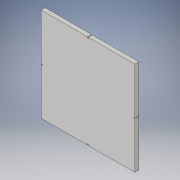
# Autodesk Inventor part: aruco_plate
Saved by Autodesk Inventor 2019 (Build 230136000, 136)
## iProperties
Created: 2024-08-28
Part Number: aruco_plate
Material: Generisch
Document SubType Name: Modeling
Designer: nic
Density: 1 g/cm^3
Appearance: Vorgabe
Author: nic
Autodesk Inventor part; units mm, degrees
ref_plane "YZ Plane" through (0, 0, 0) normal (1, 0, 0) x (0, 1, 0)
ref_plane "XZ Plane" through (0, 0, 0) normal (0, 1, 0) x (-1, 0, 0)
ref_plane "XY Plane" through (0, 0, 0) normal (0, 0, 1) x (1, 0, 0)
sketch "Skizze1" plane through (0, 0, 0) normal (0, 0, 1) x (1, 0, 0)
  line L0 (-34.5, 34.5) -> (34.5, 34.5)
  line L1 (34.5, 34.5) -> (34.5, -34.5)
  line L2 (34.5, -34.5) -> (-34.5, -34.5)
  line L3 (-34.5, -34.5) -> (-34.5, 34.5)
  line L4 (-34.5, 34.5) -> (34.5, -34.5) construction
  line L5 (34.5, 34.5) -> (-34.5, -34.5) construction
  point P0 (0, 0)
  dimension "d0" = 69
  dimension "d1" = 69
  constraints: 12 end point, 2 midpoint, 2 parallel, 1 horizontal, 1 perpendicular
  measures "d0" distance of L1.end L2.end
  measures "d1" distance of L0.end L1.end
extrude "Extrusion1" add sketch "Skizze1" along normal blind 3
sketch "Skizze2" plane through (0, 0, 0) normal (0, 0, -1) x (-1, 0, 0)
  line L0 (34.5, 34.5) -> (-34.5, 34.5) construction
  line L1 (-34.5, 34.5) -> (-34.5, -34.5) construction
  line L2 (-34.5, -34.5) -> (34.5, -34.5) construction
  line L3 (34.5, -34.5) -> (34.5, 34.5) construction
  line L4 (-0.25, -36.2092) -> (0.25, -36.2092) construction
  line L5 (0.25, -36.2092) -> (0.25, 36.2092) construction
  line L6 (0.25, 36.2092) -> (-0.25, 36.2092) construction
  line L7 (-0.25, 36.2092) -> (-0.25, -36.2092) construction
  line L8 (-0.25, -36.2092) -> (0.25, 36.2092) construction
  line L9 (0.25, -36.2092) -> (-0.25, 36.2092) construction
  line L10 (-34.5, -34.5) -> (-34.5, 34.5) construction
  line L11 (34.5, -0.25) -> (-34.5, -0.25) construction
  line L12 (-34.5, -0.25) -> (-34.5, 0.25) construction
  line L13 (-34.5, 0.25) -> (34.5, 0.25) construction
  line L14 (34.5, 0.25) -> (34.5, -0.25) construction
  line L15 (34.5, -0.25) -> (-34.5, 0.25) construction
  line L16 (-34.5, -0.25) -> (34.5, 0.25) construction
  line L17 (-0.2382, 34.5) -> (0.2313, 34.5)
  line L18 (0.2313, 34.5) -> (0.2313, 33.5)
  line L19 (0.2313, 33.5) -> (-0.2382, 33.5)
  line L20 (-0.2382, 33.5) -> (-0.2382, 34.5)
  line L21 (-34.5, 0.25) -> (-33.5, 0.25)
  line L22 (-33.5, 0.25) -> (-33.5, -0.2428)
  line L23 (-33.5, -0.2428) -> (-34.5, -0.2428)
  line L24 (-34.5, -0.2428) -> (-34.5, 0.25)
  line L25 (34.5, -34.5) -> (-34.5, -34.5) projected
  line L26 (-0.25, -34.5) -> (0.25, -34.5)
  line L27 (0.25, -34.5) -> (0.25, -33.5)
  line L28 (0.25, -33.5) -> (-0.25, -33.5)
  line L29 (-0.25, -33.5) -> (-0.25, -34.5)
  line L30 (34.5, 0.25) -> (33.5, 0.25)
  line L31 (33.5, 0.25) -> (33.5, -0.2428)
  line L32 (33.5, -0.2428) -> (34.5, -0.2428)
  line L33 (34.5, -0.2428) -> (34.5, 0.25)
  point P0 (0, 0)
  dimension "d4" = 0.5
  dimension "d5" = 0.5
  dimension "d6" = 1
  dimension "d7" = 1
  dimension "d8" = 1
  dimension "d9" = 1
  constraints: 56 end point, 12 parallel, 9 point on line, 6 horizontal, 6 perpendicular, 4 midpoint
  measures "d4" distance of L6.end L5.end
  measures "d5" distance of L11.end L12.end
  measures "d6" distance of L17.end L18.end
  measures "d7" distance of L22.end L23.end
  measures "d8" distance of L27.end L26.end
  measures "d9" distance of L32.end L31.end
extrude "Extrusion2" cut sketch "Skizze2" against normal through all
sketch "Skizze3" plane through (0, 0, 0) normal (0, 0, -1) x (-1, 0, 0)
  line L0 (13.5227, 32.2329) -> (32.4466, 32.2329) construction
  line L1 (32.4466, 32.2329) -> (32.4466, 28.5854) construction
  line L2 (32.4466, 28.5854) -> (13.5227, 28.5854) construction
  line L3 (13.5227, 28.5854) -> (13.5227, 32.2329) construction
  line L4 (14.0662, 25.0881) -> (28.9058, 25.0881) construction
  line L5 (28.9058, 25.0881) -> (28.9058, 21.4406) construction
  line L6 (28.9058, 21.4406) -> (14.0662, 21.4406) construction
  line L7 (14.0662, 21.4406) -> (14.0662, 25.0881) construction
  spline S0 degree 2 poles (16.4431, 22.6261) (16.4431, 22.3737) (16.2814, 21.9426) (16.1339, 21.7838) knots 0 0 0 1 2 2 2
  spline S1 degree 2 poles (16.1339, 21.7838) (15.9864, 21.6249) (15.5468, 21.4406) (15.2745, 21.4406) knots 0 0 0 1 2 2 2
  spline S2 degree 2 poles (15.2745, 21.4406) (15.0249, 21.4406) (14.5371, 21.5512) (14.3584, 21.6391) knots 0 0 0 1 2 2 2
  line L8 (14.3584, 21.6391) -> (14.3584, 22.1355)
  line L9 (14.3584, 22.1355) -> (14.3924, 22.1355)
  spline S3 degree 2 poles (14.3924, 22.1355) (14.4463, 22.0958) (14.6477, 21.9937) (14.7696, 21.9483) knots 0 0 0 1 2 2 2
  spline S4 degree 2 poles (14.7696, 21.9483) (14.9086, 21.9001) (15.1384, 21.8462) (15.283, 21.8462) knots 0 0 0 1 2 2 2
  spline S5 degree 2 poles (15.283, 21.8462) (15.4248, 21.8462) (15.6914, 21.9483) (15.7879, 22.0589) knots 0 0 0 1 2 2 2
  spline S6 degree 2 poles (15.7879, 22.0589) (15.8758, 22.1638) (15.9666, 22.4418) (15.9666, 22.629) knots 0 0 0 1 2 2 2
  spline S7 degree 2 poles (15.9666, 22.629) (15.9666, 22.8162) (15.8645, 23.0544) (15.768, 23.1338) knots 0 0 0 1 2 2 2
  spline S8 degree 2 poles (15.768, 23.1338) (15.6687, 23.2218) (15.3738, 23.2955) (15.1951, 23.2955) knots 0 0 0 1 2 2 2
  spline S9 degree 2 poles (15.1951, 23.2955) (15.0022, 23.2955) (14.6193, 23.236) (14.503, 23.2104) knots 0 0 0 1 2 2 2
  line L10 (14.503, 23.2104) -> (14.503, 25.0143)
  line L11 (14.503, 25.0143) -> (16.4232, 25.0143)
  line L12 (16.4232, 25.0143) -> (16.4232, 24.6031)
  line L13 (16.4232, 24.6031) -> (14.954, 24.6031)
  line L14 (14.954, 24.6031) -> (14.954, 23.6699)
  spline S10 degree 2 poles (14.954, 23.6699) (15.0391, 23.6813) (15.2036, 23.6898) (15.2717, 23.6898) knots 0 0 0 1 2 2 2
  spline S11 degree 2 poles (15.2717, 23.6898) (15.5411, 23.6898) (15.9127, 23.6018) (16.0828, 23.4714) knots 0 0 0 1 2 2 2
  spline S12 degree 2 poles (16.0828, 23.4714) (16.2559, 23.3409) (16.4431, 22.9438) (16.4431, 22.6261) knots 0 0 0 1 2 2 2
  spline S13 degree 2 poles (17.8924, 24.6825) (17.7648, 24.6825) (17.5123, 24.6201) (17.3904, 24.5719) knots 0 0 0 1 2 2 2
  spline S14 degree 2 poles (17.3904, 24.5719) (17.2769, 24.5236) (17.1096, 24.4215) (17.0444, 24.3761) knots 0 0 0 1 2 2 2
  line L15 (17.0444, 24.3761) -> (17.016, 24.3761)
  line L16 (17.016, 24.3761) -> (17.016, 24.8725)
  spline S15 degree 2 poles (17.016, 24.8725) (17.1692, 24.9548) (17.6939, 25.0881) (17.9293, 25.0881) knots 0 0 0 1 2 2 2
  spline S16 degree 2 poles (17.9293, 25.0881) (18.1675, 25.0881) (18.5221, 24.9916) (18.6667, 24.8895) knots 0 0 0 1 2 2 2
  spline S17 degree 2 poles (18.6667, 24.8895) (18.8199, 24.7789) (18.9787, 24.4584) (18.9787, 24.2428) knots 0 0 0 1 2 2 2
  spline S18 degree 2 poles (18.9787, 24.2428) (18.9787, 23.9535) (18.5986, 23.5167) (18.332, 23.46) knots 0 0 0 1 2 2 2
  line L17 (18.332, 23.46) -> (18.332, 23.426)
  spline S19 degree 2 poles (18.332, 23.426) (18.4427, 23.4033) (18.6951, 23.3012) (18.8029, 23.1991) knots 0 0 0 1 2 2 2
  spline S20 degree 2 poles (18.8029, 23.1991) (18.9106, 23.0998) (19.0468, 22.7821) (19.0468, 22.5524) knots 0 0 0 1 2 2 2
  spline S21 degree 2 poles (19.0468, 22.5524) (19.0468, 22.317) (18.8851, 21.9171) (18.7376, 21.7639) knots 0 0 0 1 2 2 2
  spline S22 degree 2 poles (18.7376, 21.7639) (18.5845, 21.6051) (18.1505, 21.4406) (17.8754, 21.4406) knots 0 0 0 1 2 2 2
  spline S23 degree 2 poles (17.8754, 21.4406) (17.6116, 21.4406) (17.0954, 21.5682) (16.9196, 21.6561) knots 0 0 0 1 2 2 2
  line L18 (16.9196, 21.6561) -> (16.9196, 22.1525)
  line L19 (16.9196, 22.1525) -> (16.9536, 22.1525)
  spline S24 degree 2 poles (16.9536, 22.1525) (17.1011, 22.0447) (17.6003, 21.8462) (17.847, 21.8462) knots 0 0 0 1 2 2 2
  spline S25 degree 2 poles (17.847, 21.8462) (17.9917, 21.8462) (18.281, 21.9369) (18.3774, 22.0419) knots 0 0 0 1 2 2 2
  spline S26 degree 2 poles (18.3774, 22.0419) (18.471, 22.1468) (18.5703, 22.3964) (18.5703, 22.5864) knots 0 0 0 1 2 2 2
  spline S27 degree 2 poles (18.5703, 22.5864) (18.5703, 22.7765) (18.4597, 23.0232) (18.3604, 23.0941) knots 0 0 0 1 2 2 2
  spline S28 degree 2 poles (18.3604, 23.0941) (18.2611, 23.165) (17.9917, 23.2189) (17.8328, 23.2189) knots 0 0 0 1 2 2 2
  line L20 (17.8328, 23.2189) -> (17.6343, 23.2189)
  line L21 (17.6343, 23.2189) -> (17.6343, 23.6075)
  line L22 (17.6343, 23.6075) -> (17.7903, 23.6075)
  spline S29 degree 2 poles (17.7903, 23.6075) (18.1051, 23.6075) (18.5022, 23.9082) (18.5022, 24.1946) knots 0 0 0 1 2 2 2
  spline S30 degree 2 poles (18.5022, 24.1946) (18.5022, 24.3279) (18.4001, 24.518) (18.3179, 24.5747) knots 0 0 0 1 2 2 2
  spline S31 degree 2 poles (18.3179, 24.5747) (18.2299, 24.6342) (18.0144, 24.6825) (17.8924, 24.6825) knots 0 0 0 1 2 2 2
  line L23 (21.6789, 21.5143) -> (21.1371, 21.5143)
  line L24 (21.1371, 21.5143) -> (20.499, 22.5013)
  line L25 (20.499, 22.5013) -> (19.8438, 21.5143)
  line L26 (19.8438, 21.5143) -> (19.3418, 21.5143)
  line L27 (19.3418, 21.5143) -> (20.2522, 22.8162)
  line L28 (20.2522, 22.8162) -> (19.3503, 24.1407)
  line L29 (19.3503, 24.1407) -> (19.892, 24.1407)
  line L30 (19.892, 24.1407) -> (20.5273, 23.1622)
  line L31 (20.5273, 23.1622) -> (21.1769, 24.1407)
  line L32 (21.1769, 24.1407) -> (21.6789, 24.1407)
  line L33 (21.6789, 24.1407) -> (20.7741, 22.8445)
  line L34 (20.7741, 22.8445) -> (21.6789, 21.5143)
  spline S32 degree 2 poles (24.0784, 22.6261) (24.0784, 22.3737) (23.9167, 21.9426) (23.7692, 21.7838) knots 0 0 0 1 2 2 2
  spline S33 degree 2 poles (23.7692, 21.7838) (23.6217, 21.6249) (23.1821, 21.4406) (22.9098, 21.4406) knots 0 0 0 1 2 2 2
  spline S34 degree 2 poles (22.9098, 21.4406) (22.6602, 21.4406) (22.1724, 21.5512) (21.9937, 21.6391) knots 0 0 0 1 2 2 2
  line L35 (21.9937, 21.6391) -> (21.9937, 22.1355)
  line L36 (21.9937, 22.1355) -> (22.0277, 22.1355)
  spline S35 degree 2 poles (22.0277, 22.1355) (22.0816, 22.0958) (22.283, 21.9937) (22.405, 21.9483) knots 0 0 0 1 2 2 2
  spline S36 degree 2 poles (22.405, 21.9483) (22.5439, 21.9001) (22.7737, 21.8462) (22.9183, 21.8462) knots 0 0 0 1 2 2 2
  spline S37 degree 2 poles (22.9183, 21.8462) (23.0602, 21.8462) (23.3268, 21.9483) (23.4232, 22.0589) knots 0 0 0 1 2 2 2
  spline S38 degree 2 poles (23.4232, 22.0589) (23.5111, 22.1638) (23.6019, 22.4418) (23.6019, 22.629) knots 0 0 0 1 2 2 2
  spline S39 degree 2 poles (23.6019, 22.629) (23.6019, 22.8162) (23.4998, 23.0544) (23.4033, 23.1338) knots 0 0 0 1 2 2 2
  spline S40 degree 2 poles (23.4033, 23.1338) (23.3041, 23.2218) (23.0091, 23.2955) (22.8304, 23.2955) knots 0 0 0 1 2 2 2
  spline S41 degree 2 poles (22.8304, 23.2955) (22.6375, 23.2955) (22.2546, 23.236) (22.1384, 23.2104) knots 0 0 0 1 2 2 2
  line L37 (22.1384, 23.2104) -> (22.1384, 25.0143)
  line L38 (22.1384, 25.0143) -> (24.0585, 25.0143)
  line L39 (24.0585, 25.0143) -> (24.0585, 24.6031)
  line L40 (24.0585, 24.6031) -> (22.5893, 24.6031)
  line L41 (22.5893, 24.6031) -> (22.5893, 23.6699)
  spline S42 degree 2 poles (22.5893, 23.6699) (22.6744, 23.6813) (22.8389, 23.6898) (22.907, 23.6898) knots 0 0 0 1 2 2 2
  spline S43 degree 2 poles (22.907, 23.6898) (23.1764, 23.6898) (23.548, 23.6018) (23.7182, 23.4714) knots 0 0 0 1 2 2 2
  spline S44 degree 2 poles (23.7182, 23.4714) (23.8912, 23.3409) (24.0784, 22.9438) (24.0784, 22.6261) knots 0 0 0 1 2 2 2
  spline S45 degree 2 poles (25.5277, 24.6825) (25.4001, 24.6825) (25.1477, 24.6201) (25.0257, 24.5719) knots 0 0 0 1 2 2 2
  spline S46 degree 2 poles (25.0257, 24.5719) (24.9123, 24.5236) (24.7449, 24.4215) (24.6797, 24.3761) knots 0 0 0 1 2 2 2
  line L42 (24.6797, 24.3761) -> (24.6513, 24.3761)
  line L43 (24.6513, 24.3761) -> (24.6513, 24.8725)
  spline S47 degree 2 poles (24.6513, 24.8725) (24.8045, 24.9548) (25.3292, 25.0881) (25.5646, 25.0881) knots 0 0 0 1 2 2 2
  spline S48 degree 2 poles (25.5646, 25.0881) (25.8029, 25.0881) (26.1574, 24.9916) (26.3021, 24.8895) knots 0 0 0 1 2 2 2
  spline S49 degree 2 poles (26.3021, 24.8895) (26.4552, 24.7789) (26.614, 24.4584) (26.614, 24.2428) knots 0 0 0 1 2 2 2
  spline S50 degree 2 poles (26.614, 24.2428) (26.614, 23.9535) (26.234, 23.5167) (25.9674, 23.46) knots 0 0 0 1 2 2 2
  line L44 (25.9674, 23.46) -> (25.9674, 23.426)
  spline S51 degree 2 poles (25.9674, 23.426) (26.078, 23.4033) (26.3304, 23.3012) (26.4382, 23.1991) knots 0 0 0 1 2 2 2
  spline S52 degree 2 poles (26.4382, 23.1991) (26.546, 23.0998) (26.6821, 22.7821) (26.6821, 22.5524) knots 0 0 0 1 2 2 2
  spline S53 degree 2 poles (26.6821, 22.5524) (26.6821, 22.317) (26.5204, 21.9171) (26.373, 21.7639) knots 0 0 0 1 2 2 2
  spline S54 degree 2 poles (26.373, 21.7639) (26.2198, 21.6051) (25.7858, 21.4406) (25.5107, 21.4406) knots 0 0 0 1 2 2 2
  spline S55 degree 2 poles (25.5107, 21.4406) (25.2469, 21.4406) (24.7307, 21.5682) (24.5549, 21.6561) knots 0 0 0 1 2 2 2
  line L45 (24.5549, 21.6561) -> (24.5549, 22.1525)
  line L46 (24.5549, 22.1525) -> (24.5889, 22.1525)
  spline S56 degree 2 poles (24.5889, 22.1525) (24.7364, 22.0447) (25.2356, 21.8462) (25.4824, 21.8462) knots 0 0 0 1 2 2 2
  spline S57 degree 2 poles (25.4824, 21.8462) (25.627, 21.8462) (25.9163, 21.9369) (26.0127, 22.0419) knots 0 0 0 1 2 2 2
  spline S58 degree 2 poles (26.0127, 22.0419) (26.1063, 22.1468) (26.2056, 22.3964) (26.2056, 22.5864) knots 0 0 0 1 2 2 2
  spline S59 degree 2 poles (26.2056, 22.5864) (26.2056, 22.7765) (26.095, 23.0232) (25.9957, 23.0941) knots 0 0 0 1 2 2 2
  spline S60 degree 2 poles (25.9957, 23.0941) (25.8965, 23.165) (25.627, 23.2189) (25.4682, 23.2189) knots 0 0 0 1 2 2 2
  line L47 (25.4682, 23.2189) -> (25.2696, 23.2189)
  line L48 (25.2696, 23.2189) -> (25.2696, 23.6075)
  line L49 (25.2696, 23.6075) -> (25.4256, 23.6075)
  spline S61 degree 2 poles (25.4256, 23.6075) (25.7405, 23.6075) (26.1375, 23.9082) (26.1375, 24.1946) knots 0 0 0 1 2 2 2
  spline S62 degree 2 poles (26.1375, 24.1946) (26.1375, 24.3279) (26.0354, 24.518) (25.9532, 24.5747) knots 0 0 0 1 2 2 2
  spline S63 degree 2 poles (25.9532, 24.5747) (25.8653, 24.6342) (25.6497, 24.6825) (25.5277, 24.6825) knots 0 0 0 1 2 2 2
  spline S64 degree 2 poles (15.9903, 29.7937) (15.9903, 29.5242) (15.8116, 29.0676) (15.6613, 28.9144) knots 0 0 0 1 2 2 2
  spline S65 degree 2 poles (15.6613, 28.9144) (15.5053, 28.7527) (15.1139, 28.5854) (14.8785, 28.5854) knots 0 0 0 1 2 2 2
  spline S66 degree 2 poles (14.8785, 28.5854) (14.6431, 28.5854) (14.2545, 28.7442) (14.107, 28.9031) knots 0 0 0 1 2 2 2
  spline S67 degree 2 poles (14.107, 28.9031) (13.9255, 29.0931) (13.7213, 29.7313) (13.7213, 30.1964) knots 0 0 0 1 2 2 2
  spline S68 degree 2 poles (13.7213, 30.1964) (13.7213, 30.6531) (13.9085, 31.3877) (14.1042, 31.66) knots 0 0 0 1 2 2 2
  spline S69 degree 2 poles (14.1042, 31.66) (14.2942, 31.9266) (14.8955, 32.2244) (15.2898, 32.2244) knots 0 0 0 1 2 2 2
  spline S70 degree 2 poles (15.2898, 32.2244) (15.406, 32.2244) (15.6103, 32.2017) (15.6868, 32.1762) knots 0 0 0 1 2 2 2
  line L50 (15.6868, 32.1762) -> (15.6868, 31.7252)
  line L51 (15.6868, 31.7252) -> (15.667, 31.7252)
  spline S71 degree 2 poles (15.667, 31.7252) (15.6018, 31.7592) (15.3635, 31.8188) (15.2274, 31.8188) knots 0 0 0 1 2 2 2
  spline S72 degree 2 poles (15.2274, 31.8188) (14.7906, 31.8188) (14.2545, 31.2288) (14.2035, 30.6502) knots 0 0 0 1 2 2 2
  spline S73 degree 2 poles (14.2035, 30.6502) (14.3708, 30.7665) (14.7225, 30.8942) (14.9324, 30.8942) knots 0 0 0 1 2 2 2
  spline S74 degree 2 poles (14.9324, 30.8942) (15.1366, 30.8942) (15.4429, 30.8119) (15.6103, 30.6871) knots 0 0 0 1 2 2 2
  spline S75 degree 2 poles (15.6103, 30.6871) (15.8031, 30.5425) (15.9903, 30.0943) (15.9903, 29.7937) knots 0 0 0 1 2 2 2
  spline S76 degree 2 poles (15.5138, 29.7738) (15.5138, 29.9894) (15.4004, 30.2815) (15.2756, 30.3836) knots 0 0 0 1 2 2 2
  spline S77 degree 2 poles (15.2756, 30.3836) (15.182, 30.4574) (14.9494, 30.5056) (14.8274, 30.5056) knots 0 0 0 1 2 2 2
  spline S78 degree 2 poles (14.8274, 30.5056) (14.6629, 30.5056) (14.3538, 30.4063) (14.2035, 30.3127) knots 0 0 0 1 2 2 2
  spline S79 degree 2 poles (14.2035, 30.3127) (14.2006, 30.2617) (14.1949, 30.1652) (14.1949, 30.0915) knots 0 0 0 1 2 2 2
  spline S80 degree 2 poles (14.1949, 30.0915) (14.1949, 29.7284) (14.3368, 29.2831) (14.4445, 29.1668) knots 0 0 0 1 2 2 2
  spline S81 degree 2 poles (14.4445, 29.1668) (14.5438, 29.0562) (14.7594, 28.9683) (14.8813, 28.9683) knots 0 0 0 1 2 2 2
  spline S82 degree 2 poles (14.8813, 28.9683) (15.165, 28.9683) (15.5138, 29.3711) (15.5138, 29.7738) knots 0 0 0 1 2 2 2
  spline S83 degree 2 poles (16.308, 31.0218) (16.308, 31.2912) (16.4838, 31.7394) (16.637, 31.901) knots 0 0 0 1 2 2 2
  spline S84 degree 2 poles (16.637, 31.901) (16.7817, 32.057) (17.2043, 32.2301) (17.4198, 32.2301) knots 0 0 0 1 2 2 2
  spline S85 degree 2 poles (17.4198, 32.2301) (17.6609, 32.2301) (18.0523, 32.0684) (18.197, 31.9152) knots 0 0 0 1 2 2 2
  spline S86 degree 2 poles (18.197, 31.9152) (18.3785, 31.7224) (18.577, 31.0984) (18.577, 30.619) knots 0 0 0 1 2 2 2
  spline S87 degree 2 poles (18.577, 30.619) (18.577, 30.1851) (18.3813, 29.4079) (18.1913, 29.1498) knots 0 0 0 1 2 2 2
  spline S88 degree 2 poles (18.1913, 29.1498) (17.9899, 28.8775) (17.4227, 28.5911) (17.0086, 28.5911) knots 0 0 0 1 2 2 2
  spline S89 degree 2 poles (17.0086, 28.5911) (16.915, 28.5911) (16.7022, 28.6109) (16.6115, 28.6393) knots 0 0 0 1 2 2 2
  line L52 (16.6115, 28.6393) -> (16.6115, 29.0903)
  line L53 (16.6115, 29.0903) -> (16.6342, 29.0903)
  spline S90 degree 2 poles (16.6342, 29.0903) (16.6937, 29.0562) (16.9433, 28.9967) (17.071, 28.9967) knots 0 0 0 1 2 2 2
  spline S91 degree 2 poles (17.071, 28.9967) (17.5304, 28.9967) (18.0552, 29.6036) (18.092, 30.1652) knots 0 0 0 1 2 2 2
  spline S92 degree 2 poles (18.092, 30.1652) (17.9048, 30.0376) (17.5645, 29.9213) (17.3631, 29.9213) knots 0 0 0 1 2 2 2
  spline S93 degree 2 poles (17.3631, 29.9213) (17.1702, 29.9213) (16.8497, 30.0064) (16.6881, 30.1284) knots 0 0 0 1 2 2 2
  spline S94 degree 2 poles (16.6881, 30.1284) (16.5009, 30.273) (16.308, 30.7126) (16.308, 31.0218) knots 0 0 0 1 2 2 2
  spline S95 degree 2 poles (18.1034, 30.724) (18.1034, 31.0785) (17.9729, 31.5267) (17.8566, 31.6486) knots 0 0 0 1 2 2 2
  spline S96 degree 2 poles (17.8566, 31.6486) (17.7545, 31.7621) (17.5418, 31.8472) (17.417, 31.8472) knots 0 0 0 1 2 2 2
  spline S97 degree 2 poles (17.417, 31.8472) (17.1277, 31.8472) (16.7845, 31.4331) (16.7845, 31.0416) knots 0 0 0 1 2 2 2
  spline S98 degree 2 poles (16.7845, 31.0416) (16.7845, 30.8204) (16.8979, 30.5339) (17.0227, 30.4318) knots 0 0 0 1 2 2 2
  spline S99 degree 2 poles (17.0227, 30.4318) (17.1135, 30.3581) (17.3376, 30.3099) (17.468, 30.3099) knots 0 0 0 1 2 2 2
  spline S100 degree 2 poles (17.468, 30.3099) (17.6184, 30.3099) (17.9644, 30.4148) (18.0949, 30.5027) knots 0 0 0 1 2 2 2
  spline S101 degree 2 poles (18.0949, 30.5027) (18.0977, 30.5368) (18.1034, 30.6531) (18.1034, 30.724) knots 0 0 0 1 2 2 2
  line L54 (21.1354, 28.6591) -> (20.5936, 28.6591)
  line L55 (20.5936, 28.6591) -> (19.9555, 29.6462)
  line L56 (19.9555, 29.6462) -> (19.3003, 28.6591)
  line L57 (19.3003, 28.6591) -> (18.7983, 28.6591)
  line L58 (18.7983, 28.6591) -> (19.7087, 29.961)
  line L59 (19.7087, 29.961) -> (18.8068, 31.2856)
  line L60 (18.8068, 31.2856) -> (19.3485, 31.2856)
  line L61 (19.3485, 31.2856) -> (19.9838, 30.307)
  line L62 (19.9838, 30.307) -> (20.6334, 31.2856)
  line L63 (20.6334, 31.2856) -> (21.1354, 31.2856)
  line L64 (21.1354, 31.2856) -> (20.2306, 29.9894)
  line L65 (20.2306, 29.9894) -> (21.1354, 28.6591)
  spline S102 degree 2 poles (23.6257, 29.7937) (23.6257, 29.5242) (23.447, 29.0676) (23.2966, 28.9144) knots 0 0 0 1 2 2 2
  spline S103 degree 2 poles (23.2966, 28.9144) (23.1406, 28.7527) (22.7492, 28.5854) (22.5138, 28.5854) knots 0 0 0 1 2 2 2
  spline S104 degree 2 poles (22.5138, 28.5854) (22.2784, 28.5854) (21.8898, 28.7442) (21.7424, 28.9031) knots 0 0 0 1 2 2 2
  spline S105 degree 2 poles (21.7424, 28.9031) (21.5608, 29.0931) (21.3566, 29.7313) (21.3566, 30.1964) knots 0 0 0 1 2 2 2
  spline S106 degree 2 poles (21.3566, 30.1964) (21.3566, 30.6531) (21.5438, 31.3877) (21.7395, 31.66) knots 0 0 0 1 2 2 2
  spline S107 degree 2 poles (21.7395, 31.66) (21.9295, 31.9266) (22.5308, 32.2244) (22.9251, 32.2244) knots 0 0 0 1 2 2 2
  spline S108 degree 2 poles (22.9251, 32.2244) (23.0414, 32.2244) (23.2456, 32.2017) (23.3222, 32.1762) knots 0 0 0 1 2 2 2
  line L66 (23.3222, 32.1762) -> (23.3222, 31.7252)
  line L67 (23.3222, 31.7252) -> (23.3023, 31.7252)
  spline S109 degree 2 poles (23.3023, 31.7252) (23.2371, 31.7592) (22.9988, 31.8188) (22.8627, 31.8188) knots 0 0 0 1 2 2 2
  spline S110 degree 2 poles (22.8627, 31.8188) (22.4259, 31.8188) (21.8898, 31.2288) (21.8388, 30.6502) knots 0 0 0 1 2 2 2
  spline S111 degree 2 poles (21.8388, 30.6502) (22.0061, 30.7665) (22.3578, 30.8942) (22.5677, 30.8942) knots 0 0 0 1 2 2 2
  spline S112 degree 2 poles (22.5677, 30.8942) (22.7719, 30.8942) (23.0783, 30.8119) (23.2456, 30.6871) knots 0 0 0 1 2 2 2
  spline S113 degree 2 poles (23.2456, 30.6871) (23.4385, 30.5425) (23.6257, 30.0943) (23.6257, 29.7937) knots 0 0 0 1 2 2 2
  spline S114 degree 2 poles (23.1492, 29.7738) (23.1492, 29.9894) (23.0357, 30.2815) (22.9109, 30.3836) knots 0 0 0 1 2 2 2
  spline S115 degree 2 poles (22.9109, 30.3836) (22.8173, 30.4574) (22.5847, 30.5056) (22.4628, 30.5056) knots 0 0 0 1 2 2 2
  spline S116 degree 2 poles (22.4628, 30.5056) (22.2983, 30.5056) (21.9891, 30.4063) (21.8388, 30.3127) knots 0 0 0 1 2 2 2
  spline S117 degree 2 poles (21.8388, 30.3127) (21.8359, 30.2617) (21.8303, 30.1652) (21.8303, 30.0915) knots 0 0 0 1 2 2 2
  spline S118 degree 2 poles (21.8303, 30.0915) (21.8303, 29.7284) (21.9721, 29.2831) (22.0799, 29.1668) knots 0 0 0 1 2 2 2
  spline S119 degree 2 poles (22.0799, 29.1668) (22.1791, 29.0562) (22.3947, 28.9683) (22.5167, 28.9683) knots 0 0 0 1 2 2 2
  spline S120 degree 2 poles (22.5167, 28.9683) (22.8003, 28.9683) (23.1492, 29.3711) (23.1492, 29.7738) knots 0 0 0 1 2 2 2
  spline S121 degree 2 poles (23.9433, 31.0218) (23.9433, 31.2912) (24.1192, 31.7394) (24.2723, 31.901) knots 0 0 0 1 2 2 2
  spline S122 degree 2 poles (24.2723, 31.901) (24.417, 32.057) (24.8396, 32.2301) (25.0552, 32.2301) knots 0 0 0 1 2 2 2
  spline S123 degree 2 poles (25.0552, 32.2301) (25.2962, 32.2301) (25.6877, 32.0684) (25.8323, 31.9152) knots 0 0 0 1 2 2 2
  spline S124 degree 2 poles (25.8323, 31.9152) (26.0138, 31.7224) (26.2124, 31.0984) (26.2124, 30.619) knots 0 0 0 1 2 2 2
  spline S125 degree 2 poles (26.2124, 30.619) (26.2124, 30.1851) (26.0167, 29.4079) (25.8266, 29.1498) knots 0 0 0 1 2 2 2
  spline S126 degree 2 poles (25.8266, 29.1498) (25.6253, 28.8775) (25.058, 28.5911) (24.6439, 28.5911) knots 0 0 0 1 2 2 2
  spline S127 degree 2 poles (24.6439, 28.5911) (24.5503, 28.5911) (24.3376, 28.6109) (24.2468, 28.6393) knots 0 0 0 1 2 2 2
  line L68 (24.2468, 28.6393) -> (24.2468, 29.0903)
  line L69 (24.2468, 29.0903) -> (24.2695, 29.0903)
  spline S128 degree 2 poles (24.2695, 29.0903) (24.3291, 29.0562) (24.5787, 28.9967) (24.7063, 28.9967) knots 0 0 0 1 2 2 2
  spline S129 degree 2 poles (24.7063, 28.9967) (25.1658, 28.9967) (25.6905, 29.6036) (25.7274, 30.1652) knots 0 0 0 1 2 2 2
  spline S130 degree 2 poles (25.7274, 30.1652) (25.5402, 30.0376) (25.1998, 29.9213) (24.9984, 29.9213) knots 0 0 0 1 2 2 2
  spline S131 degree 2 poles (24.9984, 29.9213) (24.8056, 29.9213) (24.4851, 30.0064) (24.3234, 30.1284) knots 0 0 0 1 2 2 2
  spline S132 degree 2 poles (24.3234, 30.1284) (24.1362, 30.273) (23.9433, 30.7126) (23.9433, 31.0218) knots 0 0 0 1 2 2 2
  spline S133 degree 2 poles (25.7387, 30.724) (25.7387, 31.0785) (25.6082, 31.5267) (25.4919, 31.6486) knots 0 0 0 1 2 2 2
  spline S134 degree 2 poles (25.4919, 31.6486) (25.3898, 31.7621) (25.1771, 31.8472) (25.0523, 31.8472) knots 0 0 0 1 2 2 2
  spline S135 degree 2 poles (25.0523, 31.8472) (24.763, 31.8472) (24.4198, 31.4331) (24.4198, 31.0416) knots 0 0 0 1 2 2 2
  spline S136 degree 2 poles (24.4198, 31.0416) (24.4198, 30.8204) (24.5333, 30.5339) (24.6581, 30.4318) knots 0 0 0 1 2 2 2
  spline S137 degree 2 poles (24.6581, 30.4318) (24.7488, 30.3581) (24.9729, 30.3099) (25.1034, 30.3099) knots 0 0 0 1 2 2 2
  spline S138 degree 2 poles (25.1034, 30.3099) (25.2537, 30.3099) (25.5997, 30.4148) (25.7302, 30.5027) knots 0 0 0 1 2 2 2
  spline S139 degree 2 poles (25.7302, 30.5027) (25.733, 30.5368) (25.7387, 30.6531) (25.7387, 30.724) knots 0 0 0 1 2 2 2
  line L70 (28.7707, 28.6591) -> (28.229, 28.6591)
  line L71 (28.229, 28.6591) -> (27.5908, 29.6462)
  line L72 (27.5908, 29.6462) -> (26.9356, 28.6591)
  line L73 (26.9356, 28.6591) -> (26.4336, 28.6591)
  line L74 (26.4336, 28.6591) -> (27.3441, 29.961)
  line L75 (27.3441, 29.961) -> (26.4421, 31.2856)
  line L76 (26.4421, 31.2856) -> (26.9838, 31.2856)
  line L77 (26.9838, 31.2856) -> (27.6192, 30.307)
  line L78 (27.6192, 30.307) -> (28.2687, 31.2856)
  line L79 (28.2687, 31.2856) -> (28.7707, 31.2856)
  line L80 (28.7707, 31.2856) -> (27.8659, 29.9894)
  line L81 (27.8659, 29.9894) -> (28.7707, 28.6591)
  spline S140 degree 2 poles (29.9932, 31.8273) (29.8655, 31.8273) (29.6131, 31.7649) (29.4911, 31.7167) knots 0 0 0 1 2 2 2
  spline S141 degree 2 poles (29.4911, 31.7167) (29.3777, 31.6685) (29.2103, 31.5664) (29.1451, 31.521) knots 0 0 0 1 2 2 2
  line L82 (29.1451, 31.521) -> (29.1167, 31.521)
  line L83 (29.1167, 31.521) -> (29.1167, 32.0173)
  spline S142 degree 2 poles (29.1167, 32.0173) (29.2699, 32.0996) (29.7946, 32.2329) (30.03, 32.2329) knots 0 0 0 1 2 2 2
  spline S143 degree 2 poles (30.03, 32.2329) (30.2683, 32.2329) (30.6228, 32.1365) (30.7675, 32.0343) knots 0 0 0 1 2 2 2
  spline S144 degree 2 poles (30.7675, 32.0343) (30.9206, 31.9237) (31.0795, 31.6032) (31.0795, 31.3877) knots 0 0 0 1 2 2 2
  spline S145 degree 2 poles (31.0795, 31.3877) (31.0795, 31.0984) (30.6994, 30.6616) (30.4328, 30.6049) knots 0 0 0 1 2 2 2
  line L84 (30.4328, 30.6049) -> (30.4328, 30.5708)
  spline S146 degree 2 poles (30.4328, 30.5708) (30.5434, 30.5481) (30.7958, 30.446) (30.9036, 30.3439) knots 0 0 0 1 2 2 2
  spline S147 degree 2 poles (30.9036, 30.3439) (31.0114, 30.2446) (31.1475, 29.927) (31.1475, 29.6972) knots 0 0 0 1 2 2 2
  spline S148 degree 2 poles (31.1475, 29.6972) (31.1475, 29.4618) (30.9859, 29.0619) (30.8384, 28.9087) knots 0 0 0 1 2 2 2
  spline S149 degree 2 poles (30.8384, 28.9087) (30.6852, 28.7499) (30.2513, 28.5854) (29.9761, 28.5854) knots 0 0 0 1 2 2 2
  spline S150 degree 2 poles (29.9761, 28.5854) (29.7124, 28.5854) (29.1962, 28.713) (29.0203, 28.801) knots 0 0 0 1 2 2 2
  line L85 (29.0203, 28.801) -> (29.0203, 29.2973)
  line L86 (29.0203, 29.2973) -> (29.0543, 29.2973)
  spline S151 degree 2 poles (29.0543, 29.2973) (29.2018, 29.1895) (29.701, 28.991) (29.9478, 28.991) knots 0 0 0 1 2 2 2
  spline S152 degree 2 poles (29.9478, 28.991) (30.0924, 28.991) (30.3817, 29.0818) (30.4782, 29.1867) knots 0 0 0 1 2 2 2
  spline S153 degree 2 poles (30.4782, 29.1867) (30.5718, 29.2916) (30.671, 29.5412) (30.671, 29.7313) knots 0 0 0 1 2 2 2
  spline S154 degree 2 poles (30.671, 29.7313) (30.671, 29.9213) (30.5604, 30.1681) (30.4612, 30.239) knots 0 0 0 1 2 2 2
  spline S155 degree 2 poles (30.4612, 30.239) (30.3619, 30.3099) (30.0924, 30.3638) (29.9336, 30.3638) knots 0 0 0 1 2 2 2
  line L87 (29.9336, 30.3638) -> (29.7351, 30.3638)
  line L88 (29.7351, 30.3638) -> (29.7351, 30.7523)
  line L89 (29.7351, 30.7523) -> (29.8911, 30.7523)
  spline S156 degree 2 poles (29.8911, 30.7523) (30.2059, 30.7523) (30.603, 31.053) (30.603, 31.3395) knots 0 0 0 1 2 2 2
  spline S157 degree 2 poles (30.603, 31.3395) (30.603, 31.4728) (30.5009, 31.6628) (30.4186, 31.7195) knots 0 0 0 1 2 2 2
  spline S158 degree 2 poles (30.4186, 31.7195) (30.3307, 31.7791) (30.1151, 31.8273) (29.9932, 31.8273) knots 0 0 0 1 2 2 2
  point P0 (0, 0)
  constraints: 4 other
extrude "Extrusion3" cut sketch "Skizze3" against normal blind 0.5
